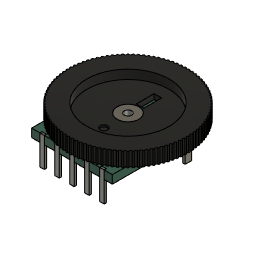
B103 volume potentiometer v3 (Autodesk Fusion 360 design; units mm, degrees)
Autodesk Fusion 360 part; units mm, degrees
note: some values were not read from the file. Chosen so that the rebuilt part matches the saved one: which bodies a step acts on; which face or edge a step refers to; the layout of a text. Set by a fixed rule: which sketch regions a step uses.
sketch "Outline" plane through (0, 0, 0) normal (0, 0, 1) x (1, 0, 0) in component "Wheel"
  circle A0 centre (0, 0) radius 7.975
  circle A1 centre (0, 0) radius 5.5
  circle A2 centre (0, 0) radius 1.45
  line L0 (-0.5, 4) -> (0.5, 4)
  line L1 (0.5, 4) -> (0.5, 1.6)
  line L2 (0.5, 1.6) -> (-0.5, 1.6)
  line L3 (-0.5, 1.6) -> (-0.5, 4)
  circle A3 centre (0.101, -3.3295) radius 0.5
  circle A4 centre (-7.975, 0) radius 0.15
  circle A5 centre (-7.9593, -0.5008) radius 0.15
  circle A6 centre (-7.9121, -0.9995) radius 0.15
  circle A7 centre (-7.8337, -1.4944) radius 0.15
  circle A8 centre (-7.7245, -1.9833) radius 0.15
  circle A9 centre (-7.5847, -2.4644) radius 0.15
  circle A10 centre (-7.415, -2.9358) radius 0.15
  circle A11 centre (-7.216, -3.3956) radius 0.15
  circle A12 centre (-6.9885, -3.842) radius 0.15
  circle A13 centre (-6.7335, -4.2732) radius 0.15
  circle A14 centre (-6.4519, -4.6876) radius 0.15
  circle A15 centre (-6.1448, -5.0835) radius 0.15
  circle A16 centre (-5.8135, -5.4593) radius 0.15
  circle A17 centre (-5.4593, -5.8135) radius 0.15
  circle A18 centre (-5.0835, -6.1448) radius 0.15
  circle A19 centre (-4.6876, -6.4519) radius 0.15
  circle A20 centre (-4.2732, -6.7335) radius 0.15
  circle A21 centre (-3.842, -6.9885) radius 0.15
  circle A22 centre (-3.3956, -7.216) radius 0.15
  circle A23 centre (-2.9358, -7.415) radius 0.15
  circle A24 centre (-2.4644, -7.5847) radius 0.15
  circle A25 centre (-1.9833, -7.7245) radius 0.15
  circle A26 centre (-1.4944, -7.8337) radius 0.15
  circle A27 centre (-0.9995, -7.9121) radius 0.15
  circle A28 centre (-0.5008, -7.9593) radius 0.15
  circle A29 centre (0, -7.975) radius 0.15
  circle A30 centre (0.5008, -7.9593) radius 0.15
  circle A31 centre (0.9995, -7.9121) radius 0.15
  circle A32 centre (1.4944, -7.8337) radius 0.15
  circle A33 centre (1.9833, -7.7245) radius 0.15
  circle A34 centre (2.4644, -7.5847) radius 0.15
  circle A35 centre (2.9358, -7.415) radius 0.15
  circle A36 centre (3.3956, -7.216) radius 0.15
  circle A37 centre (3.842, -6.9885) radius 0.15
  circle A38 centre (4.2732, -6.7335) radius 0.15
  circle A39 centre (4.6876, -6.4519) radius 0.15
  circle A40 centre (5.0835, -6.1448) radius 0.15
  circle A41 centre (5.4593, -5.8135) radius 0.15
  circle A42 centre (5.8135, -5.4593) radius 0.15
  circle A43 centre (6.1448, -5.0835) radius 0.15
  circle A44 centre (6.4519, -4.6876) radius 0.15
  circle A45 centre (6.7335, -4.2732) radius 0.15
  circle A46 centre (6.9885, -3.842) radius 0.15
  circle A47 centre (7.216, -3.3956) radius 0.15
  circle A48 centre (7.415, -2.9358) radius 0.15
  circle A49 centre (7.5847, -2.4644) radius 0.15
  circle A50 centre (7.7245, -1.9833) radius 0.15
  circle A51 centre (7.8337, -1.4944) radius 0.15
  circle A52 centre (7.9121, -0.9995) radius 0.15
  circle A53 centre (7.9593, -0.5008) radius 0.15
  circle A54 centre (7.975, 0) radius 0.15
  circle A55 centre (7.9593, 0.5008) radius 0.15
  circle A56 centre (7.9121, 0.9995) radius 0.15
  circle A57 centre (7.8337, 1.4944) radius 0.15
  circle A58 centre (7.7245, 1.9833) radius 0.15
  circle A59 centre (7.5847, 2.4644) radius 0.15
  circle A60 centre (7.415, 2.9358) radius 0.15
  circle A61 centre (7.216, 3.3956) radius 0.15
  circle A62 centre (6.9885, 3.842) radius 0.15
  circle A63 centre (6.7335, 4.2732) radius 0.15
  circle A64 centre (6.4519, 4.6876) radius 0.15
  circle A65 centre (6.1448, 5.0835) radius 0.15
  circle A66 centre (5.8135, 5.4593) radius 0.15
  circle A67 centre (5.4593, 5.8135) radius 0.15
  circle A68 centre (5.0835, 6.1448) radius 0.15
  circle A69 centre (4.6876, 6.4519) radius 0.15
  circle A70 centre (4.2732, 6.7335) radius 0.15
  circle A71 centre (3.842, 6.9885) radius 0.15
  circle A72 centre (3.3956, 7.216) radius 0.15
  circle A73 centre (2.9358, 7.415) radius 0.15
  circle A74 centre (2.4644, 7.5847) radius 0.15
  circle A75 centre (1.9833, 7.7245) radius 0.15
  circle A76 centre (1.4944, 7.8337) radius 0.15
  circle A77 centre (0.9995, 7.9121) radius 0.15
  circle A78 centre (0.5008, 7.9593) radius 0.15
  circle A79 centre (0, 7.975) radius 0.15
  circle A80 centre (-0.5008, 7.9593) radius 0.15
  circle A81 centre (-0.9995, 7.9121) radius 0.15
  circle A82 centre (-1.4944, 7.8337) radius 0.15
  circle A83 centre (-1.9833, 7.7245) radius 0.15
  circle A84 centre (-2.4644, 7.5847) radius 0.15
  circle A85 centre (-2.9358, 7.415) radius 0.15
  circle A86 centre (-3.3956, 7.216) radius 0.15
  circle A87 centre (-3.842, 6.9885) radius 0.15
  circle A88 centre (-4.2732, 6.7335) radius 0.15
  circle A89 centre (-4.6876, 6.4519) radius 0.15
  circle A90 centre (-5.0835, 6.1448) radius 0.15
  circle A91 centre (-5.4593, 5.8135) radius 0.15
  circle A92 centre (-5.8135, 5.4593) radius 0.15
  circle A93 centre (-6.1448, 5.0835) radius 0.15
  circle A94 centre (-6.4519, 4.6876) radius 0.15
  circle A95 centre (-6.7335, 4.2732) radius 0.15
  circle A96 centre (-6.9885, 3.842) radius 0.15
  circle A97 centre (-7.216, 3.3956) radius 0.15
  circle A98 centre (-7.415, 2.9358) radius 0.15
  circle A99 centre (-7.5847, 2.4644) radius 0.15
  circle A100 centre (-7.7245, 1.9833) radius 0.15
  circle A101 centre (-7.8337, 1.4944) radius 0.15
  circle A102 centre (-7.9121, 0.9995) radius 0.15
  circle A103 centre (-7.9593, 0.5008) radius 0.15
  circle A104 centre (0, 0) radius 0.5
  point P0 (0, 1.6)
  dimension "d1" = 15.95
  dimension "d2" = 11
  dimension "d3" = 2.9
  dimension "d4" = 1
  dimension "d5" = 2.4
  dimension "d6" = 1
  dimension "d7" = 4
  dimension "d8" = 0.3
  dimension "d10" = 360
  dimension "d50" = 1
  constraint coincident A0.centre A1.centre
  constraint horizontal L0
  constraint vertical L1
  constraint horizontal L2
  constraint vertical L3
  constraint midpoint L2 P0
  constraint vertical A0.centre P0
  constraint coincident A0 A4.centre
  constraint concentric A2 A104
  measures "d1" diameter of A0
  measures "d2" diameter of A1
  measures "d3" diameter of A2
  measures "d4" distance of L0.start L0.end
  measures "d5" distance of L0.start L2.end
  measures "d6" diameter of A3
  measures "d7" distance of A0.centre L0
  measures "d8" diameter of A4
  measures "d50" diameter of A104
extrude "Extrude1" add sketch "Outline" along normal blind 1.9 contours A0 A4 A5 A6 A7 A8 A9 A10 A11 A12 A13 A14 A15 A16 A17 A18 A19 A20 A21 A22 A23 A24 A25 A26 A27 A28 A29 A30 A31 A32 A33 A34 A35 A36 A37 A38 A39 A40 A41 A42 A43 A44 A45 A46 A47 A48 A49 A50 A51 A52 A53 A54 A55 A56 A57 A58 A59 A60 A61 A62 A63 A64 A65 A66 A67 A68 A69 A70 A71 A72 A73 A74 A75 A76 A77 A78 A79 A80 A81 A82 A83 A84 A85 A86 A87 A88 A89 A90 A91 A92 A93 A94 A95 A96 A97 A98 A99 A100 A101 A102 A103 makes body 1 in component "Wheel"
extrude "Extrude2" add sketch "Outline" along normal blind 0.7 contours A1 | A3 bodies 1 in component "Wheel"
sketch "Sketch1" plane through (0, 0, 0) normal (0, 0, 1) x (-1, 0, 0) in component "Board"
  line L0 (-0.5, -1.6) -> (0.5, -1.6)
  line L1 (0.5, -1.6) -> (0.5, -4)
  line L2 (0.5, -4) -> (-0.5, -4)
  line L3 (-0.5, -4) -> (-0.5, -1.6)
  circle A0 centre (0, 0) radius 1.45
  circle A1 centre (0, 0) radius 5.5
  circle A2 centre (0, 0) radius 5.4
  line L4 (-5.4, 7.5) -> (5.4, 7.5)
  line L5 (5.4, 7.5) -> (5.4, -7.5)
  line L6 (5.4, -7.5) -> (-5.4, -7.5)
  line L7 (-5.4, -7.5) -> (-5.4, 7.5)
  line L8 (-5.4, 7.5) -> (5.4, -7.5) construction
  line L9 (5.4, 7.5) -> (-5.4, -7.5) construction
  line L10 (-3.15, 3.8405) -> (3.15, 3.8405)
  line L11 (3.15, 3.8405) -> (3.15, 1.8405)
  line L12 (3.15, 1.8405) -> (-3.15, 1.8405)
  line L13 (-3.15, 1.8405) -> (-3.15, 3.8405)
  line L14 (-3.15, 3.8405) -> (3.15, 1.8405) construction
  line L15 (3.15, 3.8405) -> (-3.15, 1.8405) construction
  line L16 (-4.5, 4.5) -> (4.5, 4.5)
  line L17 (4.5, 4.5) -> (4.5, -4.5)
  line L18 (4.5, -4.5) -> (-4.5, -4.5)
  line L19 (-4.5, -4.5) -> (-4.5, 4.5)
  line L20 (-4.5, 4.5) -> (4.5, -4.5) construction
  line L21 (4.5, 4.5) -> (-4.5, -4.5) construction
  line L22 (0.3, 7.2) -> (-0.3, 7.2)
  line L23 (-0.3, 7.2) -> (-0.3, 7.5)
  line L24 (-0.3, 7.5) -> (0.3, 7.5)
  line L25 (0.3, 7.5) -> (0.3, 7.2)
  line L26 (-3.7, 7.2) -> (-4.3, 7.2)
  line L27 (-4.3, 7.2) -> (-4.3, 7.5)
  line L28 (-3.7, 7.5) -> (-3.7, 7.2)
  line L29 (-4.3, 7.5) -> (-3.7, 7.5)
  line L30 (-1.7, 7.2) -> (-2.3, 7.2)
  line L31 (-2.3, 7.2) -> (-2.3, 7.5)
  line L32 (-1.7, 7.5) -> (-1.7, 7.2)
  line L33 (-2.3, 7.5) -> (-1.7, 7.5)
  line L34 (2.3, 7.2) -> (1.7, 7.2)
  line L35 (1.7, 7.2) -> (1.7, 7.5)
  line L36 (2.3, 7.5) -> (2.3, 7.2)
  line L37 (1.7, 7.5) -> (2.3, 7.5)
  line L38 (4.3, 7.2) -> (3.7, 7.2)
  line L39 (3.7, 7.2) -> (3.7, 7.5)
  line L40 (4.3, 7.5) -> (4.3, 7.2)
  line L41 (3.7, 7.5) -> (4.3, 7.5)
  circle A3 centre (0, 5.9103) radius 0.9
  circle A4 centre (0, 5.9103) radius 0.5
  circle A5 centre (-4, 5.9103) radius 0.5
  circle A6 centre (-4, 5.9103) radius 0.9
  circle A7 centre (-2, 5.9103) radius 0.5
  circle A8 centre (-2, 5.9103) radius 0.9
  circle A9 centre (2, 5.9103) radius 0.5
  circle A10 centre (2, 5.9103) radius 0.9
  circle A11 centre (4, 5.9103) radius 0.5
  circle A12 centre (4, 5.9103) radius 0.9
  circle A13 centre (0, 0) radius 0.5
  line L42 (-5.27, -3.25) -> (-4.94, -3.25)
  line L43 (-4.94, -3.25) -> (-4.94, -2.37)
  line L44 (-4.94, -2.37) -> (-5.27, -2.37)
  line L45 (-5.27, -2.37) -> (-5.27, -3.25)
  line L46 (4.94, -2.3705) -> (5.27, -2.3705)
  line L47 (5.27, -2.3705) -> (5.27, -3.2505)
  line L48 (5.27, -3.2505) -> (4.94, -3.2505)
  line L49 (4.94, -3.2505) -> (4.94, -2.3705)
  line L50 (-4.94, -2.37) -> (4.94, -3.2505) construction
  line L51 (4.94, -2.3705) -> (-4.94, -3.25) construction
  line L52 (-4.5, 1.8405) -> (-5.4, 1.8405)
  line L53 (4.5, 1.8405) -> (5.4, 1.8405)
  line L54 (4.94, -3.2505) -> (4.3121, -3.2505)
  line L55 (5.27, -2.3705) -> (5.27, -1.1778)
  line L56 (-5.27, -2.37) -> (-5.27, -1.1778)
  line L57 (-4.94, -3.25) -> (-4.3125, -3.25)
  line L58 (-2.1874, 3.6177) -> (2.2462, 3.6177) construction
  line L59 (2.2462, 3.6177) -> (2.2462, 1.6177) construction
  line L60 (2.2462, 1.6177) -> (-2.1874, 1.6177) construction
  line L61 (-2.1874, 1.6177) -> (-2.1874, 3.6177) construction
  point P0 (0, 2.8405)
  point P1 (0, 7.2)
  point P2 (0, -2.8102)
  dimension "d15" = 10.8
  dimension "d16" = 10.8
  dimension "d17" = 15
  dimension "d18" = 6.3
  dimension "d19" = 2
  dimension "d20" = 9
  dimension "d21" = 9
  dimension "d22" = 0.6
  dimension "d23" = 0.3
  dimension "d26" = 2
  dimension "d27" = 0
  dimension "d33" = 1.8
  dimension "d34" = 1
  dimension "d37" = 2
  dimension "d38" = 0
  dimension "d46" = 1
  dimension "d53" = 0.33
  dimension "d54" = 0.88
  dimension "d55" = 0.33
  dimension "d56" = 0.88
  dimension "d57" = 9.88
  dimension "d58" = 10.75
  text T0 "B103" font "Arial" height 2 align ink ink in box 0 x 0 at (-2.1774, 3.5977) x (1, 0) y (0, -1) spacing 1 height is em
  constraint concentric A0 A2
  constraint horizontal L4
  constraint perpendicular L4 L5
  constraint parallel L4 L6
  constraint parallel L5 L7
  constraint coincident L8 A0.centre
  constraint coincident L9 A0.centre
  constraint coincident A0.centre A1.centre
  constraint horizontal L10
  constraint perpendicular L10 L11
  constraint parallel L10 L12
  constraint parallel L11 L13
  constraint coincident L14 P0
  constraint coincident L15 P0
  constraint horizontal L16
  constraint perpendicular L16 L17
  constraint parallel L16 L18
  constraint parallel L17 L19
  constraint coincident L20 A0.centre
  constraint coincident L21 A0.centre
  constraint horizontal L22
  constraint vertical L23
  constraint horizontal L24
  constraint vertical L25
  constraint collinear L4 L24
  constraint midpoint L22 P1
  constraint vertical A0.centre P1
  constraint vertical P1 A3.centre
  constraint concentric A3 A4
  constraint horizontal L42
  constraint vertical L43
  constraint horizontal L44
  constraint vertical L45
  constraint horizontal L46
  constraint vertical L47
  constraint horizontal L48
  constraint vertical L49
  constraint midpoint L51 P2
  constraint vertical A0.centre P2
  constraint coincident L19 L52.start
  constraint coincident L7 L52.end
  constraint perpendicular L7 L52
  constraint coincident L17 L53.start
  constraint coincident L5 L53.end
  constraint perpendicular L5 L53
  constraint coincident A2 L54.end
  constraint perpendicular L49 L54
  constraint coincident A2 L55.end
  constraint perpendicular L46 L55
  constraint coincident A2 L56.end
  constraint perpendicular L44 L56
  constraint coincident A2 L57.end
  constraint perpendicular L56 L57
  constraint perpendicular L58 L59
  constraint parallel L58 L60
  constraint parallel L59 L61
  measures "d15" diameter of A2
  measures "d16" distance of L5.end L6.end
  measures "d17" distance of L4.end L5.end
  measures "d18" distance of L11.end L12.end
  measures "d19" distance of L10.end L11.end
  measures "d20" distance of L17.end L18.end
  measures "d21" distance of L16.end L17.end
  measures "d22" distance of L22.start L22.end
  measures "d23" distance of L22.start L24.end
  measures "d33" diameter of A3
  measures "d34" diameter of A4
  measures "d46" diameter of A13
  measures "d53" distance of L42.start L42.end
  measures "d54" distance of L42.start L44.end
  measures "d55" distance of L46.start L46.end
  measures "d56" distance of L46.start L48.end
  measures "d57" distance of L43.end L46.start
  measures "d58" distance of L4 L42
extrude "Extrude1'" add sketch "Sketch1" against normal blind 1.1 separate body contours L0 L1 L2 L3 | A0 | A1 L5 | A1 A2 L5 L53 | A1 L5 L53 | A1 A2 L5 L55 | A1 A2 L17 L53 | A1 L4 L5 L7 L16 L17 L19 L22 L23 L25 L26 L27 L28 L30 L31 L32 L34 L35 L36 L38 L39 L40 A3 A8 A10 L52 L53 | A2 L17 L53 | A1 A2 L17 L46 L49 L55 | A1 A2 L16 L17 | A1 L16 L17 | A2 L17 L53 | A1 L46 L49 | A1 A2 L16 A10 | A2 L16 L17 L18 L19 | L4 L38 L39 L40 L41 | A1 A2 L17 L54 | A1 A2 L7 L56 | A1 L7 | A1 A2 A10 | A1 A10 | A2 L16 A3 A8 A10 | A1 A2 L18 L54 | A1 L7 L52 | A1 A2 L7 L52 | A1 A2 L19 L43 L44 L56 | A2 L19 L52 | A1 A2 A3 A10 | A2 A10 | A1 A2 L16 A8 | A1 A2 L16 L19 | L4 L34 L35 L36 L37 | A1 A2 L18 | A2 L18 | A1 A2 L19 L52 | A1 L43 L44 | A2 L19 L52 | A1 A2 A3 A4 | A1 A3 A4 | A1 A2 A8 | A2 A8 | A1 L16 L19 | A1 A2 L18 L57 | A1 A2 L19 L57 | A1 A4 | A1 A4 | A2 A3 | A1 A2 A3 A8 | A1 A8 | L4 L22 L23 L24 L25 | L4 L26 L27 L28 L29 | L4 L30 L31 L32 L33 | L10 L11 L12 L13 | A5 | A6 | A7 | A9 | A11 | A12 | A13 makes body 2 in component "Board"
extrude "Extrude2'" add sketch "Sketch1" sketch "Sketch1" against normal blind 0.2 separate body contours L0 L1 L2 L3 | A0 | A1 A2 L5 L53 | A1 L5 L53 | A1 A2 L5 L55 | A2 L17 L53 | A1 L46 L55 | A1 A2 L17 L46 L49 L55 | A1 A2 L16 L17 | A1 L16 L17 | A1 L46 L47 L48 L49 | A2 L16 L17 L18 L19 | A1 A2 L17 L54 | A1 L17 L49 L54 | A1 A2 L7 L56 | A1 A2 A10 | A1 A10 | A1 L17 L54 | A1 L7 L52 | A1 A2 L7 L52 | A1 A2 L19 L43 L44 L56 | A1 L44 L56 | A2 L19 L52 | A2 A10 | A1 A2 L16 L19 | A1 L42 L43 L44 L45 | A1 A2 A3 A4 | A1 A3 A4 | A1 A2 A8 | A2 A8 | A1 L16 L19 | A1 L19 L43 L57 | A1 A2 L19 L57 | A2 A3 | A1 A8 | A1 L19 L57 | A6 | A12 | A13 picked at (4.6099, -1.1866) picked at (-4.6099, -1.1866) of sketch 2 text T0 start surface through (0, 0, -1.1) normal (0, 0, 1) makes body 3 at (-0.995, 0.273, -1.1) makes body 4 at (-0.7615, -5.8408, -1.3) makes body 5 at (-2.7615, -5.8408, -1.3) makes body 6 at (1.2385, -5.9799, -1.1) makes body 7 at (3.2367, -5.8656, -1.1) makes body 8 at (-4.7633, -5.8656, -1.1) makes body 9 at (0.3034, -2.7198, -1.1) makes body 10 at (-0.3298, -2.9917, -1.1) makes body 11 at (-1.9055, -2.7997, -1.1) makes body 12 at (2.1142, -2.8747, -1.1) in component "Board"
extrude "Extrude3" add sketch "Sketch1" along normal blind -2.85 and the other way up to surface (-1.1 mm away) from surface at -1.1 separate body contours L4 L38 L39 L40 L41 | L4 L34 L35 L36 L37 | L4 L22 L23 L24 L25 | L4 L26 L27 L28 L29 | L4 L30 L31 L32 L33 makes body 13 at (-0.1, -7.5, -2.6333) makes body 14 at (2.1, -7.5, -1.3167) makes body 15 at (-1.9, -7.5, -1.3167) makes body 16 at (4.1, -7.2, -2.6333) makes body 17 at (-3.9, -7.2, -2.6333) in component "Board"
extrude "Extrude4" cut sketch "Sketch1" against normal up to surface (1.1 mm away) contours L4 L38 L39 L40 L41 | L4 L34 L35 L36 L37 | L4 L22 L23 L24 L25 | L4 L26 L27 L28 L29 | L4 L30 L31 L32 L33 bodies 2 in component "Board"
extrude "Extrude5" cut sketch "Sketch1" along normal blind 0.2 from surface at -1.3 contours A13 bodies 3 in component "Board"
extrude "Extrude3'" add sketch "Outline" along normal up to surface (0.7 mm away) separate body contours A2 makes body 18 in component "Wheel"
extrude "Extrude6" add sketch "Sketch1" against normal blind 2.5 from surface at -1.3 contours A1 L46 L47 L48 L49 | A1 L42 L43 L44 L45 bodies 3 in component "Board"
extrude "Extrude4'" cut sketch "Outline" against normal blind 0.25 from surface at 0.7 contours A3 bodies 1 in component "Wheel"
component "Wheel" placed x (1, 0, 0) y (0, 1, 0) z (0, 0, 1) at (0, 0, 0)
component "Board" placed x (1, 0, 0) y (0, 1, 0) z (0, 0, 1) at (0, 0, 0)
named bodies: "Wheel", "Board", "Pin"
